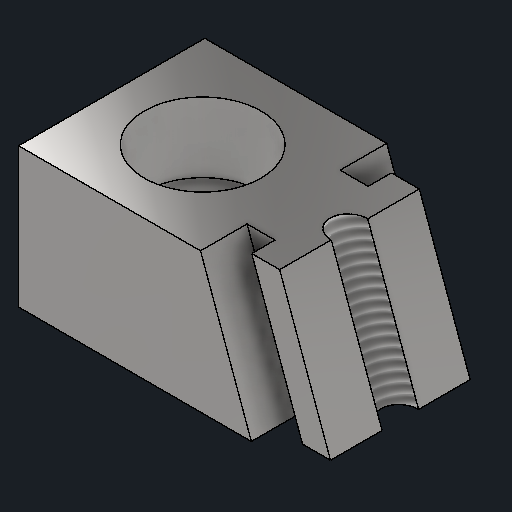
# Autodesk Inventor part: Part1
Saved by Autodesk Inventor 2026.2 (Build 302298000, 298)
## iProperties
Created: 2026-09-23
Part Number: Part1
Material: Steel, Alloy
Document SubType Name: Modeling
Designer: JoshuaEah
Density: 7.73 g/cm^3
Appearance: Semi-Polished
Author: JoshuaEah
Autodesk Inventor part; units mm, degrees
ref_plane "YZ Plane" through (0, 0, 0) normal (1, 0, 0) x (0, 1, 0)
ref_plane "XZ Plane" through (0, 0, 0) normal (0, 1, 0) x (-1, 0, 0)
sketch "Sketch1" plane through (0, 0, 0) normal (0, 1, 0) x (-1, 0, 0)
  line L0 (0, 0) -> (-39.37, 0)
  line L1 (-39.37, 0) -> (-39.37, -25.4)
  line L2 (-39.37, -25.4) -> (0, -25.4)
  line L3 (0, -25.4) -> (0, 0)
  line L4 (-35.56, -25.4) -> (-35.56, 0)
  line L5 (0, -12.7) -> (-39.37, -12.7) construction
  line L6 (-31.75, -25.4) -> (-31.75, 0)
  line L7 (-31.75, -19.05) -> (-35.56, -19.05)
  line L8 (-31.75, -6.35) -> (-35.56, -6.35)
  line L9 (-35.56, -22.225) -> (-39.37, -22.225)
  line L10 (-35.56, -3.175) -> (-39.37, -3.175)
  point P0 (-35.56, -6.35)
  point P1 (-39.37, -3.175)
  dimension "d7" = 25.4
  dimension "d10" = 3.81
  dimension "d34" = 3.81
  dimension "d35" = 12.7
  dimension "d36" = 19.05
  dimension "d37" = 31.75
  constraints: 22 end point, 8 point on line, 4 perpendicular, 4 symmetric about line, 2 horizontal, 2 midpoint, 2 parallel, 1 coincident
  measures "d7" distance of L2.end L0.start
  measures "d10" distance between parallel lines of L1 L4
  measures "d34" distance between parallel lines of L4 L6
  measures "d35" diameter of L7 L5
  measures "d36" diameter of L9 L5
  measures "d37" distance between parallel lines of L6 L3
extrude "Extrusion1" add sketch "Sketch1" along normal blind 19.05
sketch "Sketch3" plane through (0, 0, 0) normal (0, 0, 1) x (1, 0, 0)
  line L0 (0, 0) -> (39.37, 0) projected
  line L1 (39.37, 0) -> (39.37, 19.05) projected
  line L2 (0, 19.05) -> (39.37, 19.05) projected
  line L3 (0, 0) -> (0, 19.05) projected
  line L4 (24.8164, 19.05) -> (31.75, 0)
  dimension "d14" = 70
  dimension "d15" = 31.75
  constraints: 2 end point, 2 point on line
  measures "d14" angle of L0 L4
  measures "d15" distance from line of L3 L4.end
sweep "Sweep1" cut profiles "Sketch1" path "Sketch3" path curves L4 contours L6 L8 L4 L0 | L4 L10 L1 L0 | L2 L4 L7 L6 | L2 L1 L9 L4
ref_plane "Work Plane3" through (39.37, 0, 0) normal (-0.342, 0.9397, 0) x (0, 0, -1)
ref_plane "Work Plane2" through (39.37, 0, 0) normal (-0.9397, -0.342, 0) x (0, 0, -1)
sketch "Sketch5" plane through (39.37, 0, 0) normal (-0.342, 0.9397, 0) x (0, 0, -1)
  point P0 (12.7, 0)
hole "Hole2" at (39.37, 0, -12.7) direction (-0.342, 0.9397, 0) diameter 4.9784 end through all
split "Split1" plane through (39.37, 0, 0) removes the side toward (0.9397, 0.342, 0)
sketch "Sketch4" plane through (0, 19.05, 0) normal (0, 1, 0) x (1, 0, 0)
  line L0 (32.4364, 15.1892) -> (32.4364, 22.225) projected
  line L1 (32.4364, 22.225) -> (28.6264, 22.225) projected
  line L2 (28.6264, 22.225) -> (28.6264, 19.05) projected
  line L3 (28.6264, 19.05) -> (24.8164, 19.05) projected
  line L4 (24.8164, 19.05) -> (24.8164, 25.4) projected
  line L5 (24.8164, 25.4) -> (0, 25.4) projected
  line L6 (0, 25.4) -> (0, 0) projected
  line L7 (0, 0) -> (24.8164, 0) projected
  line L8 (24.8164, 0) -> (24.8164, 6.35) projected
  line L9 (24.8164, 6.35) -> (28.6264, 6.35) projected
  line L10 (28.6264, 6.35) -> (28.6264, 3.175) projected
  line L11 (28.6264, 3.175) -> (32.4364, 3.175) projected
  line L12 (32.4364, 3.175) -> (32.4364, 10.2108) projected
  ellipse E0 centre (32.4364, 12.7) end of major axis (29.7874, 12.7) minor radius 2.4892 (32.4364, 15.1892) -> (32.4364, 10.2108) ccw projected
  point P0 (12.4082, 12.7)
  point P1 (0, 12.7)
  point P2 (12.4082, 25.4)
  constraints: 2 midpoint, 1 horizontal alignment, 1 vertical alignment, 1 other
hole "Hole1" at (12.4082, 19.05, -12.7) direction (0, -1, 0) diameter 10.0838 end through all counterbore diameter 15.875 counterbore depth 9.525
equation "\"d10\" = d34"
equation "\"d34\" = slotWidth"
equation "\"d14\" = slopeAngle"
equation "\"d18\" = slopeAngle"
equation "\"slopeAngle\" = 70deg"
equation "\"slotWidth\" = 3.81"
body "Solid1"
